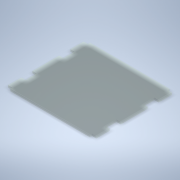
# Autodesk Inventor part: board cover
Saved by Autodesk Inventor 2022.2 (Build 262287010, 287A)
## iProperties
Created: 2021-05-28
Part Number: board cover
Material: Glass
Document SubType Name: Modeling
Designer: benka
Density: 2.18 g/cm^3
Appearance: Clear
Author: benka
Autodesk Inventor part; units mm, degrees
ref_plane "YZ Plane" through (0, 0, 0) normal (1, 0, 0) x (0, 1, 0)
ref_plane "XZ Plane" through (0, 0, 0) normal (0, 1, 0) x (-1, 0, 0)
ref_plane "XY Plane" through (0, 0, 0) normal (0, 0, 1) x (1, 0, 0)
sketch "Sketch1" plane through (0, 0, 0) normal (0, 1, 0) x (-1, 0, 0)
  line L0 (-94, -88.7502) -> (-94, -93.7502) projected
  line L1 (-104, -88.7502) -> (-94, -88.7502) projected
  line L2 (-104, -57.5002) -> (-104, -88.7502) projected
  line L3 (-94, -57.5002) -> (-104, -57.5002) projected
  line L4 (-94, -31.2502) -> (-94, -57.5002) projected
  line L5 (-104, -31.2502) -> (-94, -31.2502) projected
  line L6 (-104, 31.7498) -> (-104, -31.2502) projected
  line L7 (-94, 31.7498) -> (-104, 31.7498) projected
  line L8 (-94, 57.9998) -> (-94, 31.7498) projected
  line L9 (-104, 57.9998) -> (-94, 57.9998) projected
  line L10 (-104, 89.2498) -> (-104, 57.9998) projected
  line L11 (-94, 89.2498) -> (-104, 89.2498) projected
  line L12 (-94, 94.2498) -> (-94, 89.2498) projected
  line L13 (94, 89.2498) -> (94, 94.2498) projected
  line L14 (104, 89.2498) -> (94, 89.2498) projected
  line L15 (104, 57.9998) -> (104, 89.2498) projected
  line L16 (94, 57.9998) -> (104, 57.9998) projected
  line L17 (94, 31.7498) -> (94, 57.9998) projected
  line L18 (104, 31.7498) -> (94, 31.7498) projected
  line L19 (104, -31.2502) -> (104, 31.7498) projected
  line L20 (94, -31.2502) -> (104, -31.2502) projected
  line L21 (94, -57.5002) -> (94, -31.2502) projected
  line L22 (104, -57.5002) -> (94, -57.5002) projected
  line L23 (104, -88.7502) -> (104, -57.5002) projected
  line L24 (94, -88.7502) -> (104, -88.7502) projected
  line L25 (94, -93.7502) -> (94, -88.7502) projected
  line L26 (-94, -93.7502) -> (94, -93.7502)
  line L27 (94, 94.2498) -> (-94, 94.2498)
  dimension "d2" = 188
  dimension "d3" = 188
  dimension "d4" = 208
  constraints: 4 end point, 1 horizontal, 1 parallel
  measures "d2" distance between parallel lines of L26 L27
  measures "d3" distance between parallel lines of L8 L17
  measures "d4" distance between parallel lines of L10 L15
extrude "Extrusion1" add sketch "Sketch1" along normal blind 5
body "Solid1"
